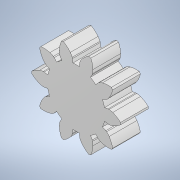
# Autodesk Inventor part: 初段多段z10
Saved by Autodesk Inventor 2022.2 (Build 262287010, 287A)
## iProperties
Created: 2022-03-13
Part Number: 初段多段z10
Material: Aluminum 2014-T6
Document SubType Name: Modeling
Designer: acps
Density: 2.78927 g/cm^3
Appearance: Satin
Author: acps
Autodesk Inventor part; units mm, degrees
ref_plane "YZ Plane" through (0, 0, 0) normal (1, 0, 0) x (0, 1, 0)
ref_plane "XZ Plane" through (0, 0, 0) normal (0, 1, 0) x (-1, 0, 0)
ref_plane "XY Plane" through (0, 0, 0) normal (0, 0, 1) x (1, 0, 0)
sketch "Sketch2" plane through (0, 0, 0) normal (0, 0, 1) x (1, 0, 0)
  arc A0 (0.5654, 4.8151) -> (0.5233, 4.6692) centre (1.183, 4.5576) ccw
  arc A1 (0.8384, 5.2827) -> (0.5654, 4.8151) centre (2.3139, 4.1079) ccw
  arc A2 (1.8376, 6.1366) -> (0.8384, 5.2827) centre (3.5373, 3.1361) ccw
  arc A3 (-2.3728, 4.2278) -> (-2.3212, 4.0851) centre (-1.7218, 4.3826) ccw
  arc A4 (-2.4268, 4.7666) -> (-2.3728, 4.2278) centre (-0.5425, 4.6834) ccw
  arc A5 (-2.1204, 6.0447) -> (-2.4268, 4.7666) centre (1.0184, 4.6164) ccw
  arc A6 (-4.4047, 2.0257) -> (-4.279, 1.9405) centre (-3.969, 2.5335) ccw
  arc A7 (-4.7651, 2.4298) -> (-4.4047, 2.0257) centre (-3.1918, 3.4701) ccw
  arc A8 (-5.2684, 3.644) -> (-4.7651, 2.4298) centre (-1.8896, 4.3333) ccw
  arc A9 (-4.7541, -0.9502) -> (-4.6024, -0.9452) centre (-4.7001, -0.2833) ccw
  arc A10 (-5.2812, -0.8359) -> (-4.7541, -0.9502) centre (-4.6219, 0.9313) ccw
  arc A11 (-6.4041, -0.1487) -> (-5.2812, -0.8359) centre (-4.0757, 2.3951) ccw
  arc A12 (-3.2876, -3.5631) -> (-3.1678, -3.4699) centre (-3.636, -2.9918) ccw
  arc A13 (-3.7833, -3.781) -> (-3.2876, -3.5631) centre (-4.2866, -1.9632) ccw
  arc A14 (-5.0936, -3.8845) -> (-3.7833, -3.781) centre (-4.7051, -0.458) ccw
  arc A15 (-0.5654, -4.8151) -> (-0.5233, -4.6692) centre (-1.183, -4.5576) ccw
  arc A16 (-0.8384, -5.2827) -> (-0.5654, -4.8151) centre (-2.3139, -4.1079) ccw
  arc A17 (-1.8376, -6.1366) -> (-0.8384, -5.2827) centre (-3.5373, -3.1361) ccw
  arc A18 (2.3728, -4.2278) -> (2.3212, -4.0851) centre (1.7218, -4.3826) ccw
  arc A19 (2.4268, -4.7666) -> (2.3728, -4.2278) centre (0.5425, -4.6834) ccw
  arc A20 (2.1204, -6.0447) -> (2.4268, -4.7666) centre (-1.0184, -4.6164) ccw
  arc A21 (4.4047, -2.0257) -> (4.279, -1.9405) centre (3.969, -2.5335) ccw
  arc A22 (4.7651, -2.4298) -> (4.4047, -2.0257) centre (3.1918, -3.4701) ccw
  arc A23 (5.2684, -3.644) -> (4.7651, -2.4298) centre (1.8896, -4.3333) ccw
  arc A24 (4.7541, 0.9502) -> (4.6024, 0.9452) centre (4.7001, 0.2833) ccw
  arc A25 (5.2832, 0.8351) -> (4.7541, 0.9502) centre (4.6219, -0.9313) ccw
  arc A26 (6.4041, 0.1487) -> (5.2832, 0.8351) centre (4.0757, -2.3951) ccw
  arc A27 (3.2876, 3.5631) -> (3.1678, 3.4699) centre (3.636, 2.9918) ccw
  arc A28 (3.7833, 3.781) -> (3.2876, 3.5631) centre (4.2866, 1.9632) ccw
  arc A29 (5.0936, 3.8845) -> (3.7833, 3.781) centre (4.7051, 0.458) ccw
  arc A30 (-0.5233, 4.6692) -> (-0.5654, 4.8151) centre (-1.183, 4.5576) ccw
  arc A31 (-0.5654, 4.8151) -> (-0.8384, 5.2827) centre (-2.3139, 4.1079) ccw
  arc A32 (-0.8384, 5.2827) -> (-1.8376, 6.1366) centre (-3.5373, 3.1361) ccw
  arc A33 (-3.1678, 3.4699) -> (-3.2876, 3.5631) centre (-3.636, 2.9918) ccw
  arc A34 (-3.2876, 3.5631) -> (-3.7833, 3.781) centre (-4.2866, 1.9632) ccw
  arc A35 (-3.7833, 3.781) -> (-5.0936, 3.8845) centre (-4.7051, 0.458) ccw
  arc A36 (-4.6024, 0.9452) -> (-4.7541, 0.9502) centre (-4.7001, 0.2833) ccw
  arc A37 (-4.7541, 0.9502) -> (-5.2832, 0.8351) centre (-4.6219, -0.9313) ccw
  arc A38 (-5.2832, 0.8351) -> (-6.4041, 0.1487) centre (-4.0757, -2.3951) ccw
  arc A39 (-4.279, -1.9405) -> (-4.4047, -2.0257) centre (-3.969, -2.5335) ccw
  arc A40 (-4.4047, -2.0257) -> (-4.7651, -2.4298) centre (-3.1918, -3.4701) ccw
  arc A41 (-4.7651, -2.4298) -> (-5.2684, -3.644) centre (-1.8896, -4.3333) ccw
  arc A42 (-2.3212, -4.0851) -> (-2.3728, -4.2278) centre (-1.7218, -4.3826) ccw
  arc A43 (-2.3728, -4.2278) -> (-2.4268, -4.7666) centre (-0.5425, -4.6834) ccw
  arc A44 (-2.4268, -4.7666) -> (-2.1204, -6.0447) centre (1.0184, -4.6164) ccw
  arc A45 (0.5233, -4.6692) -> (0.5654, -4.8151) centre (1.183, -4.5576) ccw
  arc A46 (0.5654, -4.8151) -> (0.8384, -5.2827) centre (2.3139, -4.1079) ccw
  arc A47 (0.8384, -5.2827) -> (1.8376, -6.1366) centre (3.5373, -3.1361) ccw
  arc A48 (3.1678, -3.4699) -> (3.2876, -3.5631) centre (3.636, -2.9918) ccw
  arc A49 (3.2876, -3.5631) -> (3.7833, -3.781) centre (4.2866, -1.9632) ccw
  arc A50 (3.7833, -3.781) -> (5.0936, -3.8845) centre (4.7051, -0.458) ccw
  arc A51 (4.6024, -0.9452) -> (4.7541, -0.9502) centre (4.7001, -0.2833) ccw
  arc A52 (4.7541, -0.9502) -> (5.2832, -0.8351) centre (4.6219, 0.9313) ccw
  arc A53 (5.2832, -0.8351) -> (6.4041, -0.1487) centre (4.0757, 2.3951) ccw
  arc A54 (4.279, 1.9405) -> (4.4047, 2.0257) centre (3.969, 2.5335) ccw
  arc A55 (4.4047, 2.0257) -> (4.7651, 2.4298) centre (3.1918, 3.4701) ccw
  arc A56 (4.7651, 2.4298) -> (5.2684, 3.644) centre (1.8896, 4.3333) ccw
  arc A57 (2.3212, 4.0851) -> (2.3728, 4.2278) centre (1.7218, 4.3826) ccw
  arc A58 (2.3728, 4.2278) -> (2.4268, 4.7666) centre (0.5425, 4.6834) ccw
  arc A59 (2.4268, 4.7666) -> (2.1204, 6.0447) centre (-1.0184, 4.6164) ccw
  arc A60 (0.4644, 4.1441) -> (-0.4644, 4.1441) centre (0, 0) ccw
  arc A61 (-2.0601, 3.6256) -> (-2.8115, 3.0796) centre (0, 0) ccw
  arc A62 (-3.7977, 1.7223) -> (-4.0847, 0.8389) centre (0, 0) ccw
  arc A63 (-4.0847, -0.8389) -> (-3.7977, -1.7223) centre (0, 0) ccw
  arc A64 (-2.8115, -3.0796) -> (-2.0601, -3.6256) centre (0, 0) ccw
  arc A65 (-0.4644, -4.1441) -> (0.4644, -4.1441) centre (0, 0) ccw
  arc A66 (2.0601, -3.6256) -> (2.8115, -3.0796) centre (0, 0) ccw
  arc A67 (3.7977, -1.7223) -> (4.0847, -0.8389) centre (0, 0) ccw
  arc A68 (4.0847, 0.8389) -> (3.7977, 1.7223) centre (0, 0) ccw
  arc A69 (2.8115, 3.0796) -> (2.0601, 3.6256) centre (0, 0) ccw
  arc A70 (-1.8376, 6.1366) -> (-2.1204, 6.0447) centre (0, 0) ccw
  arc A71 (-5.0936, 3.8845) -> (-5.2684, 3.644) centre (0, 0) ccw
  arc A72 (-6.4041, 0.1487) -> (-6.4041, -0.1487) centre (0, 0) ccw
  arc A73 (-5.2684, -3.644) -> (-5.0936, -3.8845) centre (0, 0) ccw
  arc A74 (-2.1204, -6.0447) -> (-1.8376, -6.1366) centre (0, 0) ccw
  arc A75 (1.8376, -6.1366) -> (2.1204, -6.0447) centre (0, 0) ccw
  arc A76 (5.0936, -3.8845) -> (5.2684, -3.644) centre (0, 0) ccw
  arc A77 (6.4041, -0.1487) -> (6.4041, 0.1487) centre (0, 0) ccw
  arc A78 (5.2684, 3.644) -> (5.0936, 3.8845) centre (0, 0) ccw
  arc A79 (2.1204, 6.0447) -> (1.8376, 6.1366) centre (0, 0) ccw
  line L0 (0.4644, 4.1441) -> (0.5233, 4.6692)
  line L1 (-2.0601, 3.6256) -> (-2.3212, 4.0851)
  line L2 (-3.7977, 1.7223) -> (-4.279, 1.9405)
  line L3 (-4.0847, -0.8389) -> (-4.6024, -0.9452)
  line L4 (-2.8115, -3.0796) -> (-3.1678, -3.4699)
  line L5 (-0.4644, -4.1441) -> (-0.5233, -4.6692)
  line L6 (2.0601, -3.6256) -> (2.3212, -4.0851)
  line L7 (3.7977, -1.7223) -> (4.279, -1.9405)
  line L8 (4.0847, 0.8389) -> (4.6024, 0.9452)
  line L9 (2.8115, 3.0796) -> (3.1678, 3.4699)
  line L10 (-0.4644, 4.1441) -> (-0.5233, 4.6692)
  line L11 (-2.8115, 3.0796) -> (-3.1678, 3.4699)
  line L12 (-4.0847, 0.8389) -> (-4.6024, 0.9452)
  line L13 (-3.7977, -1.7223) -> (-4.279, -1.9405)
  line L14 (-2.0601, -3.6256) -> (-2.3212, -4.0851)
  line L15 (0.4644, -4.1441) -> (0.5233, -4.6692)
  line L16 (2.8115, -3.0796) -> (3.1678, -3.4699)
  line L17 (4.0847, -0.8389) -> (4.6024, -0.9452)
  line L18 (3.7977, 1.7223) -> (4.279, 1.9405)
  line L19 (2.0601, 3.6256) -> (2.3212, 4.0851)
  point P0 (0, 0)
  constraints: 160 point on circle, 80 centre point, 40 end point
extrude "Extrusion1" add sketch "Sketch2" against normal blind 4
body "Solid1"
